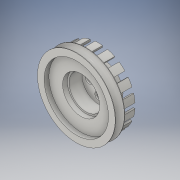
# Autodesk Inventor part: wheel
Saved by Autodesk Inventor 2016 (Build 200138000, 138)
## iProperties
Created: 2016-02-13
Part Number: wheel
Material: PC/ABS Plastic
Document SubType Name: Modeling
Designer: jforce
Density: 0.357273 g/cm^3
Appearance: Smooth - White
Author: jforce
## iProperties of the stored document wheel_3DPrint.ipt
Created: 2016-02-16
Part Number: wheel_3DPrint
Material: Generic
Document SubType Name: Modeling
Designer: jforce
Density: 1 g/cm^3
Appearance: Default
Author: jforce
Autodesk Inventor part; units mm, degrees
ref_plane "YZ Plane" through (0, 0, 0) normal (1, 0, 0) x (0, 1, 0)
ref_plane "XZ Plane" through (0, 0, 0) normal (0, 1, 0) x (-1, 0, 0)
ref_plane "XY Plane" through (0, 0, 0) normal (0, 0, 1) x (1, 0, 0)
sketch "Sketch1" plane through (0, 0, 0) normal (0, 0, 1) x (1, 0, 0)
  circle A0 centre (0, 0) radius 12
  dimension "d0" = 24
  constraints: 1 centre point, 1 coincident
  measures "d0" diameter of A0
extrude "Extrusion1" add sketch "Sketch1" along normal blind 3
sketch "Sketch2" plane through (0, 0, 3) normal (0, 0, 1) x (1, 0, 0)
  circle A0 centre (0, 0) radius 10.5
  circle A1 centre (0, 0) radius 12
  dimension "d3" = 21
  dimension "d4" = 24
  constraints: 2 centre point, 2 coincident
  measures "d3" diameter of A0
  measures "d4" diameter of A1
extrude "Extrusion2" add sketch "Sketch2" along normal blind 8
sketch "Sketch3" plane through (0, 0, 11) normal (0, 0, 1) x (1, 0, 0)
  circle A0 centre (0, 0) radius 11.5166
  circle A1 centre (0, 0) radius 24.13
  dimension "d7" = 48.26
  constraints: 2 centre point, 2 coincident
  measures "d7" diameter of A1
extrude "Extrusion3" add sketch "Sketch3" along normal blind 3
sketch "Sketch4" plane through (0, 0, 3) normal (0, 0, 1) x (1, 0, 0)
  line L0 (0, 0) -> (0, -6) construction
  dimension "d10" = 6
  constraints: 2 end point, 1 vertical
  measures "d10" distance of L0.start L0.end
hole "Hole1" at (0, -6, 3) direction (0, 0, -1) diameter 4 depth 3 tip angle 118 counterbore diameter 5 counterbore depth 0.85
pattern_circular "Circular Pattern1" count 4 over 360 about axis through (0, 0, -10) along (0, 0, 1) of "Hole1"
sketch "Sketch5" plane through (0, 0, 14) normal (0, 0, 1) x (1, 0, 0)
  circle A0 centre (0, 0) radius 24.13
  circle A1 centre (0, 0) radius 20
  dimension "d21" = 40
  dimension "d35" = 48.26
  constraints: 2 centre point, 2 coincident
  measures "d21" diameter of A1
  measures "d35" diameter of A0
extrude "Extrusion4" add sketch "Sketch5" along normal blind 3
sketch "Sketch6" plane through (0, 0, 0) normal (1, 0, 0) x (0, 1, 0)
  line L0 (-24.13, 11) -> (24.13, 11) projected
  line L1 (24.13, 17) -> (-24.13, 17) projected
  line L2 (0, -3.4) -> (0, 20.4) projected
  line L3 (24.13, 11) -> (24.13, 17) projected
  line L4 (24.13, 11) -> (24.13, 17) projected
  circle A0 centre (24.13, 14) radius 2.7
  point P0 (0, 0)
  point P1 (-22, 14)
  point P2 (-22.067, 14)
  dimension "d36" = 5.4
  constraints: 1 centre point, 1 midpoint
  measures "d36" diameter of A0
revolve "Revolution1" cut sketch "Sketch6" angle 360 about axis through (0, 0, -10) along (0, 0, 1) contours A0 L3 | L3 A0
sketch "Sketch7" plane through (0, 0, 11) normal (0, 0, -1) x (-1, 0, 0)
  circle A0 centre (0, 0) radius 12 projected
  line L0 (0, 0) -> (29.1463, 0) construction
  line L1 (0, 0) -> (28.4807, 0) construction
  arc A1 (2.2343, 21.2579) -> (-2.2343, 21.2579) centre (0, 0) ccw
  arc A2 (2.3519, 22.3767) -> (-2.3519, 22.3767) centre (0, 0) ccw
  line L2 (-2.2343, 21.2579) -> (-2.3519, 22.3767)
  line L3 (2.2343, 21.2579) -> (2.3519, 22.3767)
  dimension "d28" = 45
  constraints: 8 end point, 4 point on circle, 2 centre point, 2 coincident, 2 horizontal
  measures "d28" diameter of A2
extrude "Extrusion5" add sketch "Sketch7" along normal blind 8 contours A1 L2 A2 L3
fillet "Fillet1" radius 1 2 edges at (0, 22.5, 11) (0, 21.375, 11)
pattern_circular "Circular Pattern2" count 18 over 360 about axis through (0, 0, -10) along (0, 0, 1) of "Extrusion5", "Fillet1"
body "Solid1"
